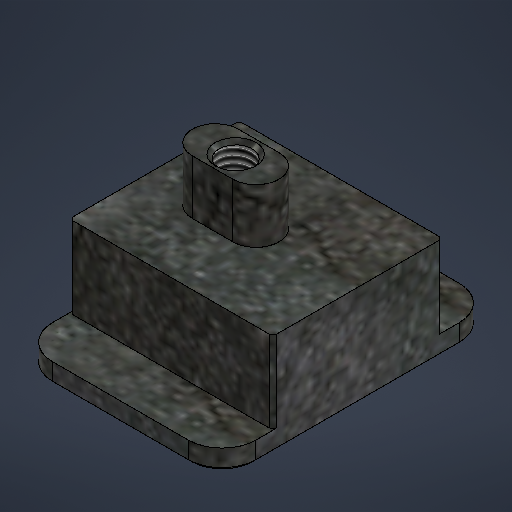
# Autodesk Inventor part: TCSM1-003
Saved by Autodesk Inventor 2025.3 (Build 293356000, 356)
## iProperties
Created: 2025-08-24
Part Number: TCSM1-003
Material: Steel
Document SubType Name: Modeling
Designer: fablabadmin
Density: 7.85 g/cm^3
Appearance: Plate
Author: fablabadmin
Autodesk Inventor part; units mm, degrees
ref_plane "YZ Plane" through (0, 0, 0) normal (1, 0, 0) x (0, 1, 0)
ref_plane "XZ Plane" through (0, 0, 0) normal (0, 1, 0) x (-1, 0, 0)
ref_plane "XY Plane" through (0, 0, 0) normal (0, 0, 1) x (1, 0, 0)
sketch "Sketch1" plane through (0, 0, 0) normal (0, 1, 0) x (-1, 0, 0)
  line L0 (15, 20) -> (-15, 20)
  line L1 (-15, 20) -> (-15, -20)
  line L2 (-15, -20) -> (15, -20)
  line L3 (15, -20) -> (15, 20)
  line L4 (15, 20) -> (-15, -20) construction
  line L5 (-15, 20) -> (15, -20) construction
  line L6 (21, 0) -> (-21, 0) construction
  line L7 (0, -28) -> (0, 28) construction
  line L8 (6, 0) -> (0, 0) construction
  line L9 (6, 3.4) -> (0, 3.4)
  line L10 (0, -3.4) -> (6, -3.4)
  arc A0 (6, -3.4) -> (6, 3.4) centre (6, 0) ccw
  arc A1 (0, 3.4) -> (0, -3.4) centre (0, 0) ccw
  line L11 (-15, 12.5) -> (15, 12.5)
  line L12 (-15, -12.5) -> (15, -12.5)
  point P0 (0, 0)
  point P1 (3, 0)
  point P2 (3, 0)
  point P3 (15, -12.5)
  dimension "d0" = 40
  dimension "d1" = 30
  dimension "d2" = 6
  dimension "d3" = 6.8
  dimension "d19" = 3
  dimension "d35" = 25
  constraints: 24 end point, 4 midpoint, 4 point on circle, 4 tangent, 3 parallel, 3 point on line, 2 centre point, 2 perpendicular, 2 symmetric about line, 1 coincident, 1 horizontal
  measures "d0" distance of L2.end L0.start
  measures "d1" distance of L1.end L2.end
  measures "d2" distance of L8.end L8.start
  measures "d3" distance between parallel lines of L9 L10
  measures "d19" distance of point (0, 0) point (3, 0)
  measures "d35" distance between parallel lines of L12 L11
extrude "Extrusion1" add sketch "Sketch1" against normal blind 23 contours L3 L11 L1 L0 | L3 L12 L1 L11 | L3 L2 L1 L12 | A0 L10 A1 L9
extrude "Extrusion2" cut sketch "Sketch1" against normal blind 8
sketch "Sketch3" plane through (0, -23, 0) normal (0, -1, 0) x (1, 0, 0)
  circle A0 centre (0, 0) radius 7.5
  dimension "d29" = 15
  constraints: 1 centre point, 1 coincident
  measures "d29" diameter of A0
extrude "Extrusion5" cut sketch "Sketch3" against normal blind 10
extrude "Extrusion6" cut sketch "Sketch1" against normal blind 20 contours L3 L11 L1 L0 | L3 L2 L1 L12
hole "Hole1" at (-3, 0, 0) direction (0, -1, 0) diameter 4.917 depth 13 countersink diameter 6 countersink angle 90 thread size "M6x1" class "6H" standard "ISO Metric profile"
fillet "Fillet1" radius 5 4 edges at (-15, -21.5, 20) (-15, -21.5, -20) (15, -21.5, -20) (15, -21.5, 20)
chamfer "Chamfer1" distance 0.5 angle 45 13 edges at (0, -23, 20) (-13.5355, -23, 18.5355) (-15, -23, 0) (-13.5355, -23, -18.5355) (0, -23, -20) (13.5355, -23, -18.5355) (15, -23, 0) (13.5355, -23, 18.5355) (-7.5, -23, 0) (-15, -14, 12.5) (-15, -14, -12.5) (15, -14, -12.5) (15, -14, 12.5)
equation "\"d4\" = slotTabH + sheetT"
equation "\"d6\" = slotTabH"
equation "\"slotTabH\" = 8"
equation "\"sheetT\" = 15"
body "Solid1"
